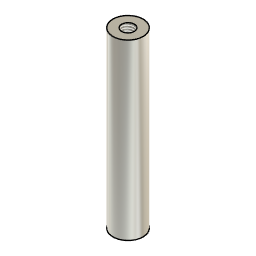
Aluminum Bar φ12 x 69.0mm (Autodesk Fusion 360 design; units mm, degrees)
Autodesk Fusion 360 part; units mm, degrees
sketch "スケッチ1" plane through (0, 0, 0) normal (0, 0, 1) x (1, 0, 0)
  circle A0 centre (0, 0) radius 6
  dimension "d1" = 12
  constraint coincident A0.centre origin
  measures "d1" diameter of A0
extrude "押し出し1" add sketch "スケッチ1" along normal blind 69
cylinder "円柱プリミティブ1" cut diameter 6 height -15 placed x (1, 0, 0) y (0, 1, 0) z (0, 0, 1) at (0, 0, 69)
thread "ねじ1" "ISO Metric profile 6.0 M6x1 6H" major diameter 6.147 minor diameter 5.035 pitch 1 angle 60 resizes the face on face at (2.9851, -0.2987, 59)
cylinder "円柱プリミティブ2" cut diameter 6 height -15 placed x (0, 1, 0) y (1, 0, 0) z (0, 0, -1) at (0, 0, 0)
thread "ねじ2" "ISO Metric profile 6.0 M6x1 6H" major diameter 6.147 minor diameter 5.035 pitch 1 angle 60 resizes the face on face at (-0.2987, 2.9851, 10)
